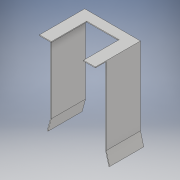
# Autodesk Inventor part: U-Part Gen 2
Saved by Autodesk Inventor 2019 (Build 230136000, 136)
## iProperties
Created: 2019-10-05
Part Number: U-Part Gen 2
Material: Generic
Document SubType Name: Modeling
Designer: Delta
Density: 1 g/cm^3
Appearance: Default
Author: Delta
Autodesk Inventor part; units mm, degrees
ref_plane "YZ Plane" through (0, 0, 0) normal (1, 0, 0) x (0, 1, 0)
ref_plane "XZ Plane" through (0, 0, 0) normal (0, 1, 0) x (-1, 0, 0)
sketch "Sketch1" plane through (0, 0, 0) normal (0, 0, 1) x (1, 0, 0)
  line L0 (0, 0) -> (109.855, 0)
  line L1 (109.855, 0) -> (109.855, -1.5875)
  line L2 (109.855, -1.5875) -> (0, -1.5875)
  line L3 (0, -1.5875) -> (0, 0)
  line L4 (109.855, 0) -> (108.2675, 0)
  line L5 (108.2675, 0) -> (108.2675, -153.2655)
  line L6 (108.2675, -153.2655) -> (109.855, -153.2655)
  line L7 (109.855, -153.2655) -> (109.855, 0)
  line L8 (0, 0) -> (1.5875, 0)
  line L9 (1.5875, 0) -> (1.5875, -153.2655)
  line L10 (1.5875, -153.2655) -> (0, -153.2655)
  line L11 (0, -153.2655) -> (0, 0)
  line L12 (0, -151.678) -> (25.4, -151.678) construction
  line L13 (1.5875, -153.2655) -> (38.1, -153.2655) construction
  line L14 (0, -153.2655) -> (-6.4677, -177.4031)
  line L15 (1.5875, -153.2655) -> (-4.9865, -177.8)
  line L16 (-6.4677, -177.4031) -> (-4.9865, -177.8)
  line L17 (54.9275, 0) -> (54.9275, -59.745)
  line L18 (109.855, -153.2655) -> (116.3227, -177.4031)
  line L19 (108.2675, -153.2655) -> (114.8415, -177.8)
  line L20 (116.3227, -177.4031) -> (114.8415, -177.8)
  dimension "d1" = 1.5875
  dimension "d2" = 1.5875
  dimension "d3" = 153.2655
  dimension "d5" = 153.2655
  dimension "d6" = 1.5875
  dimension "d13" = 1.5875
  dimension "d15" = 106.68
  dimension "d28" = 0
  dimension "d29" = 75
  dimension "d30" = 25.4
  dimension "d31" = 53.34
  dimension "d32" = 177.8
  dimension "d33" = 24.5345
  constraints: 42 end point, 6 parallel, 5 horizontal, 4 perpendicular, 2 symmetric about line, 1 midpoint, 1 point on line, 1 vertical
  measures "d1" distance of L0.end L1.end
  measures "d2" distance of L6.end L5.end
  measures "d3" distance of L5.end L4.end
  measures "d5" distance between parallel lines of L10 L0
  measures "d6" distance of L12.start L10.end
  measures "d13" distance between parallel lines of L11 L9
  measures "d15" distance between parallel lines of L5 L9
  measures "d28" angle of L14 L15
  measures "d29" angle of L10 L15
  measures "d30" distance from line of L9.end L16
  measures "d31" distance between parallel lines of L5 L17
  measures "d32" distance from line of L0 L15.end
  measures "d33" distance from line of L10 L15.end
extrude "Extrusion4" add sketch "Sketch1" along normal blind 88.9 contours L0 L9 L2 L3 | L0 L17 L2 L9 | L0 L5 L2 L17 | L0 L1 L2 L5
extrude "Extrusion5" add sketch "Sketch1" along normal blind 67.31 contours L0 L9 L2 L3 | L2 L9 L10 L11 | L10 L15 L16 L14 | L0 L1 L2 L5 | L2 L7 L6 L5 | L6 L18 L20 L19
ref_plane "Work Plane3" through (54.9275, 0, 88.9) normal (1, 0, 0) x (0, 0, -1)
sketch "Sketch4" plane through (0, 0, 0) normal (0, 1, 0) x (1, 0, 0)
  line L0 (0, -88.9) -> (109.855, -88.9) projected
  line L1 (23.1775, -88.9) -> (86.6775, -88.9)
  line L2 (86.6775, -88.9) -> (86.6775, -19.05)
  line L3 (86.6775, -19.05) -> (23.1775, -19.05)
  line L4 (23.1775, -19.05) -> (23.1775, -88.9)
  line L5 (109.855, 0) -> (109.855, -88.9) projected
  line L6 (0, 0) -> (0, -88.9) projected
  line L7 (109.855, 0) -> (0, 0) projected
  dimension "d42" = 109.855
  dimension "d43" = 63.5
  dimension "d44" = 23.1775
  dimension "d45" = 19.05
  constraints: 8 end point, 2 parallel, 1 horizontal, 1 perpendicular, 1 point on line
  measures "d42" distance between parallel lines of L5 L6
  measures "d43" distance of L2.end L3.end
  measures "d44" distance between parallel lines of L4 L6
  measures "d45" distance between parallel lines of L7 L3
extrude "Extrusion7" cut sketch "Sketch4" against normal through all contours L4 L3 L2 L0
equation "\"d2\" = d1"
equation "\"d3\" = d5"
equation "\"d6\" = d4"
equation "\"d13\" = d2"
equation "\"d44\" = -0.5 * d43 + 0.5 * d42"
equation "\"d4\" = d2"
body "Solid2"
